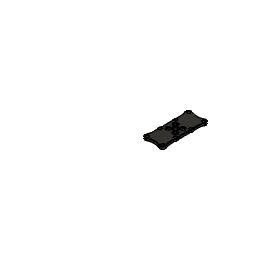
Long BattPad (Autodesk Fusion 360 design; units mm, degrees)
Autodesk Fusion 360 part; units mm, degrees
sketch "Sketch1" plane through (0, 0, 11) normal (0, 0, 1) x (-1, 0, 0)
  circle A0 centre (-10, -10) radius 1.6
  line L0 (-1.822921, 0.176777) -> (-0.176777, 1.822921)
  arc A1 (0.176777, 1.822921) -> (-0.176777, 1.822921) centre (0, 1.646145) ccw
  line L1 (0.176777, 1.822921) -> (1.822921, 0.176777)
  arc A2 (1.822921, -0.176777) -> (1.822921, 0.176777) centre (1.646145, 0) ccw
  line L2 (1.822921, -0.176777) -> (0.176777, -1.822921)
  arc A3 (-0.176777, -1.822921) -> (0.176777, -1.822921) centre (0, -1.646145) ccw
  line L3 (-0.176777, -1.822921) -> (-1.822921, -0.176777)
  arc A4 (-1.822921, 0.176777) -> (-1.822921, -0.176777) centre (-1.646145, 0) ccw
  circle A5 centre (10, 10) radius 1.6
  circle A6 centre (10, -27) radius 1.6
  line L4 (-5.126603, 7.5) -> (-3.5, 7.5)
  arc A7 (-2.5, 6.5) -> (-3.5, 7.5) centre (-3.5, 6.5) ccw
  line L5 (-2.5, 6.5) -> (-2.5, 3.5)
  arc A8 (-3.5, 2.5) -> (-2.5, 3.5) centre (-3.5, 3.5) ccw
  line L6 (-3.5, 2.5) -> (-6.5, 2.5)
  arc A9 (-7.5, 3.5) -> (-6.5, 2.5) centre (-6.5, 3.5) ccw
  line L7 (-7.5, 3.5) -> (-7.5, 5.126603)
  arc A10 (-7.083333, 5.938836) -> (-7.5, 5.126603) centre (-6.5, 5.126603) ccw
  arc A11 (-7.083333, 5.938836) -> (-5.938836, 7.083333) centre (-10, 10) ccw
  arc A12 (-5.126603, 7.5) -> (-5.938836, 7.083333) centre (-5.126603, 6.5) ccw
  circle A13 centre (10, -10) radius 1.6
  circle A14 centre (-10, 10) radius 1.6
  circle A15 centre (-10, -27) radius 1.6
  line L8 (-7.5, -5.126603) -> (-7.5, -3.5)
  arc A16 (-6.5, -2.5) -> (-7.5, -3.5) centre (-6.5, -3.5) ccw
  line L9 (-6.5, -2.5) -> (-3.5, -2.5)
  arc A17 (-2.5, -3.5) -> (-3.5, -2.5) centre (-3.5, -3.5) ccw
  line L10 (-2.5, -3.5) -> (-2.5, -6.5)
  arc A18 (-3.5, -7.5) -> (-2.5, -6.5) centre (-3.5, -6.5) ccw
  line L11 (-3.5, -7.5) -> (-5.126603, -7.5)
  arc A19 (-5.938836, -7.083333) -> (-5.126603, -7.5) centre (-5.126603, -6.5) ccw
  arc A20 (-5.938836, -7.083333) -> (-7.083333, -5.938836) centre (-10, -10) ccw
  arc A21 (-7.5, -5.126603) -> (-7.083333, -5.938836) centre (-6.5, -5.126603) ccw
  circle A22 centre (-10, 27) radius 1.6
  line L12 (5.126603, -7.5) -> (3.5, -7.5)
  arc A23 (2.5, -6.5) -> (3.5, -7.5) centre (3.5, -6.5) ccw
  line L13 (2.5, -6.5) -> (2.5, -3.5)
  arc A24 (3.5, -2.5) -> (2.5, -3.5) centre (3.5, -3.5) ccw
  line L14 (3.5, -2.5) -> (6.5, -2.5)
  arc A25 (7.5, -3.5) -> (6.5, -2.5) centre (6.5, -3.5) ccw
  line L15 (7.5, -3.5) -> (7.5, -5.126603)
  arc A26 (7.083333, -5.938836) -> (7.5, -5.126603) centre (6.5, -5.126603) ccw
  arc A27 (7.083333, -5.938836) -> (5.938836, -7.083333) centre (10, -10) ccw
  arc A28 (5.126603, -7.5) -> (5.938836, -7.083333) centre (5.126603, -6.5) ccw
  line L16 (7.5, 5.126603) -> (7.5, 3.5)
  arc A29 (6.5, 2.5) -> (7.5, 3.5) centre (6.5, 3.5) ccw
  line L17 (6.5, 2.5) -> (3.5, 2.5)
  arc A30 (2.5, 3.5) -> (3.5, 2.5) centre (3.5, 3.5) ccw
  line L18 (2.5, 3.5) -> (2.5, 6.5)
  arc A31 (3.5, 7.5) -> (2.5, 6.5) centre (3.5, 6.5) ccw
  line L19 (3.5, 7.5) -> (5.126603, 7.5)
  arc A32 (5.938836, 7.083333) -> (5.126603, 7.5) centre (5.126603, 6.5) ccw
  arc A33 (5.938836, 7.083333) -> (7.083333, 5.938836) centre (10, 10) ccw
  arc A34 (7.5, 5.126603) -> (7.083333, 5.938836) centre (6.5, 5.126603) ccw
  circle A35 centre (10, 27) radius 1.6
  line L20 (-11.749994, -13.807897) -> (-11.749994, -17.591692)
  arc A36 (-13.425731, -25.474592) -> (-11.749994, -17.591692) centre (-31.128994, -17.591692) ccw
  arc A37 (-13.425731, -25.474592) -> (-8.378659, -30.381383) centre (-10, -27) ccw
  arc A38 (8.378659, -30.381383) -> (-8.378659, -30.381383) centre (0, -47.85547) ccw
  arc A39 (8.378659, -30.381383) -> (13.425731, -25.474592) centre (10, -27) ccw
  arc A40 (11.749994, -17.591692) -> (13.425731, -25.474592) centre (31.128994, -17.591692) ccw
  line L21 (11.749994, -17.591692) -> (11.749994, -13.807897)
  arc A41 (12.395159, -11.351189) -> (11.749994, -13.807897) centre (16.749994, -13.807897) ccw
  arc A42 (12.395159, -11.351189) -> (12.395159, -8.648811) centre (10, -10) ccw
  arc A43 (11.749994, -6.192103) -> (12.395159, -8.648811) centre (16.749994, -6.192103) ccw
  line L22 (11.749994, -6.192103) -> (11.749994, 6.192103)
  arc A44 (12.395159, 8.648811) -> (11.749994, 6.192103) centre (16.749994, 6.192103) ccw
  arc A45 (12.395159, 8.648811) -> (12.395159, 11.351189) centre (10, 10) ccw
  arc A46 (11.749994, 13.807897) -> (12.395159, 11.351189) centre (16.749994, 13.807897) ccw
  line L23 (11.749994, 13.807897) -> (11.749994, 17.591692)
  arc A47 (13.425731, 25.474592) -> (11.749994, 17.591692) centre (31.128994, 17.591692) ccw
  arc A48 (13.425731, 25.474592) -> (8.378659, 30.381383) centre (10, 27) ccw
  arc A49 (-8.378659, 30.381383) -> (8.378659, 30.381383) centre (0, 47.85547) ccw
  arc A50 (-8.378659, 30.381383) -> (-13.425731, 25.474592) centre (-10, 27) ccw
  arc A51 (-11.749994, 17.591692) -> (-13.425731, 25.474592) centre (-31.128994, 17.591692) ccw
  line L24 (-11.749994, 17.591692) -> (-11.749994, 13.807897)
  arc A52 (-12.395159, 11.351189) -> (-11.749994, 13.807897) centre (-16.749994, 13.807897) ccw
  arc A53 (-12.395159, 11.351189) -> (-12.395159, 8.648811) centre (-10, 10) ccw
  arc A54 (-11.749994, 6.192103) -> (-12.395159, 8.648811) centre (-16.749994, 6.192103) ccw
  line L25 (-11.749994, 6.192103) -> (-11.749994, -6.192103)
  arc A55 (-12.395159, -8.648811) -> (-11.749994, -6.192103) centre (-16.749994, -6.192103) ccw
  arc A56 (-12.395159, -8.648811) -> (-12.395159, -11.351189) centre (-10, -10) ccw
  arc A57 (-11.749994, -13.807897) -> (-12.395159, -11.351189) centre (-16.749994, -13.807897) ccw
  arc A58 (-13.06032, -25.637302) -> (-8.551602, -30.020702) centre (-10, -27) ccw
  arc A59 (8.551602, -30.020702) -> (-8.551602, -30.020702) centre (0, -47.85547) ccw
  arc A60 (8.551602, -30.020702) -> (13.06032, -25.637302) centre (10, -27) ccw
  arc A61 (11.349994, -17.591692) -> (13.06032, -25.637302) centre (31.128994, -17.591692) ccw
  line L26 (11.349994, -17.591692) -> (11.349994, -13.807897)
  arc A62 (12.046772, -11.154653) -> (11.349994, -13.807897) centre (16.749994, -13.807897) ccw
  arc A63 (12.046772, -11.154653) -> (12.046772, -8.845347) centre (10, -10) ccw
  arc A64 (11.349994, -6.192103) -> (12.046772, -8.845347) centre (16.749994, -6.192103) ccw
  line L27 (11.349994, -6.192103) -> (11.349994, 6.192103)
  arc A65 (12.046772, 8.845347) -> (11.349994, 6.192103) centre (16.749994, 6.192103) ccw
  arc A66 (12.046772, 8.845347) -> (12.046772, 11.154653) centre (10, 10) ccw
  arc A67 (11.349994, 13.807897) -> (12.046772, 11.154653) centre (16.749994, 13.807897) ccw
  line L28 (11.349994, 13.807897) -> (11.349994, 17.591692)
  arc A68 (13.06032, 25.637302) -> (11.349994, 17.591692) centre (31.128994, 17.591692) ccw
  arc A69 (13.06032, 25.637302) -> (8.551602, 30.020702) centre (10, 27) ccw
  arc A70 (-8.551602, 30.020702) -> (8.551602, 30.020702) centre (0, 47.85547) ccw
  arc A71 (-8.551602, 30.020702) -> (-13.06032, 25.637302) centre (-10, 27) ccw
  arc A72 (-11.349994, 17.591692) -> (-13.06032, 25.637302) centre (-31.128994, 17.591692) ccw
  line L29 (-11.349994, 17.591692) -> (-11.349994, 13.807897)
  arc A73 (-12.046772, 11.154653) -> (-11.349994, 13.807897) centre (-16.749994, 13.807897) ccw
  arc A74 (-12.046772, 11.154653) -> (-12.046772, 8.845347) centre (-10, 10) ccw
  arc A75 (-11.349994, 6.192103) -> (-12.046772, 8.845347) centre (-16.749994, 6.192103) ccw
  line L30 (-11.349994, 6.192103) -> (-11.349994, -6.192103)
  arc A76 (-12.046772, -8.845347) -> (-11.349994, -6.192103) centre (-16.749994, -6.192103) ccw
  arc A77 (-12.046772, -8.845347) -> (-12.046772, -11.154653) centre (-10, -10) ccw
  arc A78 (-11.349994, -13.807897) -> (-12.046772, -11.154653) centre (-16.749994, -13.807897) ccw
  line L31 (-11.349994, -13.807897) -> (-11.349994, -17.591692)
  arc A79 (-13.06032, -25.637302) -> (-11.349994, -17.591692) centre (-31.128994, -17.591692) ccw
  circle A80 centre (-10, 10) radius 1.8
  circle A81 centre (10, 10) radius 1.8
  circle A82 centre (10, -10) radius 1.8
  circle A83 centre (10, -27) radius 1.8
  circle A84 centre (-10, -27) radius 1.8
  circle A85 centre (-10, 27) radius 1.8
  circle A86 centre (10, 27) radius 1.8
  dimension "d510" = 0.4
  dimension "d511" = 0.2
  dimension "d512" = 0.2
  dimension "d513" = 0.2
  dimension "d514" = 0.2
  dimension "d515" = 0.2
  dimension "d516" = 0.2
  dimension "d517" = 0.2
extrude "Extrude1" add sketch "Sketch1" along normal blind 3 contours A58 A59 A60 A61 L26 A62 A63 A64 L27 A65 A66 A67 L28 A68 A69 A70 A71 A72 L29 A73 A74 A75 L30 A76 A77 A78 L31 A79 picked at (0, 14.331819)
fillet "Fillet1" radius 0.336 28 edges at (11.7823, -21.704388, 14) (11.349994, -15.699795, 14) (11.527093, -12.436292, 14) (12.35, -10, 14) (11.527093, -7.563708, 14) (11.349994, 0, 14) (11.527093, 7.563708, 14) (12.35, 10, 14) (11.527093, 12.436292, 14) (11.349994, 15.699795, 14) (11.7823, 21.704388, 14) (12.335192, 29.401953, 14) (0, 28.07647, 14) (-12.335192, 29.401953, 14) (-11.7823, 21.704388, 14) (-11.349994, 15.699795, 14) (-11.527093, 12.436292, 14) (-12.35, 10, 14) (-11.527093, 7.563708, 14) (-11.349994, 0, 14) (-11.527093, -7.563708, 14) (-12.35, -10, 14) (-11.527093, -12.436292, 14) (-11.349994, -15.699795, 14) (-11.7823, -21.704388, 14) (-12.335192, -29.401953, 14) (0, -28.07647, 14) (12.335192, -29.401953, 14)
fillet "Fillet2" radius 0.4 56 edges at (4.313301, 7.5, 14) (5.583038, 7.389757, 14) (6.464466, 6.464466, 14) (7.389757, 5.583038, 14) (7.5, 4.313301, 14) (7.207107, 2.792893, 14) (5, 2.5, 14) (2.792893, 2.792893, 14) (2.5, 5, 14) (2.792893, 7.207107, 14) (7.5, -4.313301, 14) (7.389757, -5.583038, 14) (6.464466, -6.464466, 14) (5.583038, -7.389757, 14) (4.313301, -7.5, 14) (2.792893, -7.207107, 14) (2.5, -5, 14) (2.792893, -2.792893, 14) (5, -2.5, 14) (7.207107, -2.792893, 14) (0, -1.896145, 14) (-0.999849, -0.999849, 14) (-1.896145, 0, 14) (-0.999849, 0.999849, 14) (0, 1.896145, 14) (0.999849, 0.999849, 14) (1.896145, 0, 14) (0.999849, -0.999849, 14) (-2.792893, -7.207107, 14) (-4.313301, -7.5, 14) (-5.583038, -7.389757, 14) (-6.464466, -6.464466, 14) (-7.389757, -5.583038, 14) (-7.5, -4.313301, 14) (-7.207107, -2.792893, 14) (-5, -2.5, 14) (-2.792893, -2.792893, 14) (-2.5, -5, 14) (-7.5, 4.313301, 14) (-7.389757, 5.583038, 14) (-6.464466, 6.464466, 14) (-5.583038, 7.389757, 14) (-4.313301, 7.5, 14) (-2.792893, 7.207107, 14) (-2.5, 5, 14) (-2.792893, 2.792893, 14) (-5, 2.5, 14) (-7.207107, 2.792893, 14) (-8.321811, 9.349092, 14) (-8.321811, -10.650908, 14) (11.678189, -10.650908, 14) (11.678189, -27.650908, 14) (-8.321811, -27.650908, 14) (11.678189, 26.349092, 14) (11.491724, 9.421415, 14) (-8.321811, 26.349092, 14)
sketch "Sketch1 (1)" plane through (0, 0, 14) normal (0, 0, 1) x (-1, 0, 0)
  circle A0 centre (-10, -10) radius 2
  circle A1 centre (10, 27) radius 2.2
  arc A2 (-11.424764, 8.323681) -> (-11.424764, 11.676319) centre (-10, 10) ccw
  arc A3 (-11.013994, 6.192103) -> (-11.424764, 8.323681) centre (-16.749994, 6.192103) ccw
  line L0 (-11.013994, 6.192103) -> (-11.013994, -6.192103)
  arc A4 (-11.754127, -9.010438) -> (-11.013994, -6.192103) centre (-16.749994, -6.192103) ccw
  arc A5 (-11.754127, -9.010438) -> (-11.754127, -10.989562) centre (-10, -10) ccw
  arc A6 (-11.013994, -13.807897) -> (-11.754127, -10.989562) centre (-16.749994, -13.807897) ccw
  line L1 (-11.013994, -13.807897) -> (-11.013994, -17.591692)
  arc A7 (-12.753374, -25.773979) -> (-11.013994, -17.591692) centre (-31.128994, -17.591692) ccw
  arc A8 (-12.753374, -25.773979) -> (-8.696874, -29.71773) centre (-10, -27) ccw
  arc A9 (8.696874, -29.71773) -> (-8.696874, -29.71773) centre (0, -47.85547) ccw
  arc A10 (8.696874, -29.71773) -> (12.753374, -25.773979) centre (10, -27) ccw
  arc A11 (11.013994, -17.591692) -> (12.753374, -25.773979) centre (31.128994, -17.591692) ccw
  line L2 (11.013994, -17.591692) -> (11.013994, -13.807897)
  arc A12 (11.424764, -11.676319) -> (11.013994, -13.807897) centre (16.749994, -13.807897) ccw
  arc A13 (11.424764, -8.323681) -> (11.424764, -11.676319) centre (10, -10) ccw
  arc A14 (11.013994, -6.192103) -> (11.424764, -8.323681) centre (16.749994, -6.192103) ccw
  line L3 (11.013994, -6.192103) -> (11.013994, 6.192103)
  arc A15 (11.424764, 8.323681) -> (11.013994, 6.192103) centre (16.749994, 6.192103) ccw
  arc A16 (11.424764, 11.676319) -> (11.424764, 8.323681) centre (10, 10) ccw
  arc A17 (11.013994, 13.807897) -> (11.424764, 11.676319) centre (16.749994, 13.807897) ccw
  line L4 (11.013994, 13.807897) -> (11.013994, 17.591692)
  arc A18 (12.753374, 25.773979) -> (11.013994, 17.591692) centre (31.128994, 17.591692) ccw
  arc A19 (12.753374, 25.773979) -> (8.696874, 29.71773) centre (10, 27) ccw
  arc A20 (-8.696874, 29.71773) -> (8.696874, 29.71773) centre (0, 47.85547) ccw
  arc A21 (-8.696874, 29.71773) -> (-12.753374, 25.773979) centre (-10, 27) ccw
  arc A22 (-11.013994, 17.591692) -> (-12.753374, 25.773979) centre (-31.128994, 17.591692) ccw
  line L5 (-11.013994, 17.591692) -> (-11.013994, 13.807897)
  arc A23 (-11.424764, 11.676319) -> (-11.013994, 13.807897) centre (-16.749994, 13.807897) ccw
  arc A24 (3.5, 7.9) -> (2.1, 6.5) centre (3.5, 6.5) ccw
  line L6 (3.5, 7.9) -> (5.126603, 7.9)
  arc A25 (6.263729, 7.316667) -> (5.126603, 7.9) centre (5.126603, 6.5) ccw
  arc A26 (6.263729, 7.316667) -> (7.316667, 6.263729) centre (10, 10) ccw
  arc A27 (7.9, 5.126603) -> (7.316667, 6.263729) centre (6.5, 5.126603) ccw
  line L7 (7.9, 5.126603) -> (7.9, 3.5)
  arc A28 (6.5, 2.1) -> (7.9, 3.5) centre (6.5, 3.5) ccw
  line L8 (6.5, 2.1) -> (3.5, 2.1)
  arc A29 (2.1, 3.5) -> (3.5, 2.1) centre (3.5, 3.5) ccw
  line L9 (2.1, 3.5) -> (2.1, 6.5)
  line L10 (-7.9, 3.5) -> (-7.9, 5.126603)
  arc A30 (-7.316667, 6.263729) -> (-7.9, 5.126603) centre (-6.5, 5.126603) ccw
  arc A31 (-7.316667, 6.263729) -> (-6.263729, 7.316667) centre (-10, 10) ccw
  arc A32 (-5.126603, 7.9) -> (-6.263729, 7.316667) centre (-5.126603, 6.5) ccw
  line L11 (-5.126603, 7.9) -> (-3.5, 7.9)
  arc A33 (-2.1, 6.5) -> (-3.5, 7.9) centre (-3.5, 6.5) ccw
  line L12 (-2.1, 6.5) -> (-2.1, 3.5)
  arc A34 (-3.5, 2.1) -> (-2.1, 3.5) centre (-3.5, 3.5) ccw
  line L13 (-3.5, 2.1) -> (-6.5, 2.1)
  arc A35 (-7.9, 3.5) -> (-6.5, 2.1) centre (-6.5, 3.5) ccw
  line L14 (-3.5, -7.9) -> (-5.126603, -7.9)
  arc A36 (-6.263729, -7.316667) -> (-5.126603, -7.9) centre (-5.126603, -6.5) ccw
  arc A37 (-6.263729, -7.316667) -> (-7.316667, -6.263729) centre (-10, -10) ccw
  arc A38 (-7.9, -5.126603) -> (-7.316667, -6.263729) centre (-6.5, -5.126603) ccw
  line L15 (-7.9, -5.126603) -> (-7.9, -3.5)
  arc A39 (-6.5, -2.1) -> (-7.9, -3.5) centre (-6.5, -3.5) ccw
  line L16 (-6.5, -2.1) -> (-3.5, -2.1)
  arc A40 (-2.1, -3.5) -> (-3.5, -2.1) centre (-3.5, -3.5) ccw
  line L17 (-2.1, -3.5) -> (-2.1, -6.5)
  arc A41 (-3.5, -7.9) -> (-2.1, -6.5) centre (-3.5, -6.5) ccw
  arc A42 (0.459619, 2.105764) -> (-0.459619, 2.105764) centre (0, 1.646145) ccw
  line L18 (0.459619, 2.105764) -> (2.105764, 0.459619)
  arc A43 (2.105764, -0.459619) -> (2.105764, 0.459619) centre (1.646145, 0) ccw
  line L19 (2.105764, -0.459619) -> (0.459619, -2.105764)
  arc A44 (-0.459619, -2.105764) -> (0.459619, -2.105764) centre (0, -1.646145) ccw
  line L20 (-0.459619, -2.105764) -> (-2.105764, -0.459619)
  arc A45 (-2.105764, 0.459619) -> (-2.105764, -0.459619) centre (-1.646145, 0) ccw
  line L21 (-2.105764, 0.459619) -> (-0.459619, 2.105764)
  line L22 (7.9, -3.5) -> (7.9, -5.126603)
  arc A46 (7.316667, -6.263729) -> (7.9, -5.126603) centre (6.5, -5.126603) ccw
  arc A47 (7.316667, -6.263729) -> (6.263729, -7.316667) centre (10, -10) ccw
  arc A48 (5.126603, -7.9) -> (6.263729, -7.316667) centre (5.126603, -6.5) ccw
  line L23 (5.126603, -7.9) -> (3.5, -7.9)
  arc A49 (2.1, -6.5) -> (3.5, -7.9) centre (3.5, -6.5) ccw
  line L24 (2.1, -6.5) -> (2.1, -3.5)
  arc A50 (3.5, -2.1) -> (2.1, -3.5) centre (3.5, -3.5) ccw
  line L25 (3.5, -2.1) -> (6.5, -2.1)
  arc A51 (7.9, -3.5) -> (6.5, -2.1) centre (6.5, -3.5) ccw
  circle A52 centre (-10, 27) radius 2.2
  circle A53 centre (-10, -27) radius 2.2
  circle A54 centre (10, -27) radius 2.2
  arc A55 (0.792893, -3.262742) -> (1.146447, -3.116295) centre (0.792893, -2.762742) ccw
  line L26 (1.146447, -3.116295) -> (3.116295, -1.146447)
  arc A56 (3.116295, -1.146447) -> (3.262742, -0.792893) centre (2.762742, -0.792893) ccw
  line L27 (3.262742, -0.792893) -> (3.262742, 0.792893)
  arc A57 (3.262742, 0.792893) -> (3.116295, 1.146447) centre (2.762742, 0.792893) ccw
  line L28 (3.116295, 1.146447) -> (1.146447, 3.116295)
  arc A58 (1.146447, 3.116295) -> (0.792893, 3.262742) centre (0.792893, 2.762742) ccw
  line L29 (0.792893, 3.262742) -> (-0.792893, 3.262742)
  arc A59 (-0.792893, 3.262742) -> (-1.146447, 3.116295) centre (-0.792893, 2.762742) ccw
  line L30 (-1.146447, 3.116295) -> (-3.116295, 1.146447)
  arc A60 (-3.116295, 1.146447) -> (-3.262742, 0.792893) centre (-2.762742, 0.792893) ccw
  line L31 (-3.262742, 0.792893) -> (-3.262742, -0.792893)
  arc A61 (-3.262742, -0.792893) -> (-3.116295, -1.146447) centre (-2.762742, -0.792893) ccw
  line L32 (-3.116295, -1.146447) -> (-1.146447, -3.116295)
  arc A62 (-1.146447, -3.116295) -> (-0.792893, -3.262742) centre (-0.792893, -2.762742) ccw
  line L33 (-0.792893, -3.262742) -> (0.792893, -3.262742)
  line L34 (3.292742, -0.792893) -> (3.292742, 0.792893)
  arc A63 (3.292742, 0.792893) -> (3.137508, 1.16766) centre (2.762742, 0.792893) ccw
  line L35 (3.137508, 1.16766) -> (1.16766, 3.137508)
  arc A64 (1.16766, 3.137508) -> (0.792893, 3.292742) centre (0.792893, 2.762742) ccw
  line L36 (0.792893, 3.292742) -> (-0.792893, 3.292742)
  arc A65 (-0.792893, 3.292742) -> (-1.16766, 3.137508) centre (-0.792893, 2.762742) ccw
  line L37 (-1.16766, 3.137508) -> (-3.137508, 1.16766)
  arc A66 (-3.137508, 1.16766) -> (-3.292742, 0.792893) centre (-2.762742, 0.792893) ccw
  line L38 (-3.292742, 0.792893) -> (-3.292742, -0.792893)
  arc A67 (-3.292742, -0.792893) -> (-3.137508, -1.16766) centre (-2.762742, -0.792893) ccw
  line L39 (-3.137508, -1.16766) -> (-1.16766, -3.137508)
  arc A68 (-1.16766, -3.137508) -> (-0.792893, -3.292742) centre (-0.792893, -2.762742) ccw
  line L40 (-0.792893, -3.292742) -> (0.792893, -3.292742)
  arc A69 (0.792893, -3.292742) -> (1.16766, -3.137508) centre (0.792893, -2.762742) ccw
  line L41 (1.16766, -3.137508) -> (3.137508, -1.16766)
  arc A70 (3.137508, -1.16766) -> (3.292742, -0.792893) centre (2.762742, -0.792893) ccw
  dimension "d584" = 0.03
extrude "Extrude2" cut sketch "Sketch1 (1)" against normal up to surface (11.5 mm away) contours A42 L18 A43 L19 A44 L20 A45 L21 | A55 L26 A56 L27 A57 L28 A58 L29 A59 L30 A60 L31 A61 L32 A62 L33 picked at (-0.701921, 0.153206) picked at (1.57412, 2.122835)
fillet "Fillet3" radius 0.4 16 edges at (-3.262742, 0, 14) (-3.224681, 0.984235, 14) (-2.131371, 2.131371, 14) (-0.984235, 3.224681, 14) (0, 3.262742, 14) (0.984235, 3.224681, 14) (2.131371, 2.131371, 14) (3.224681, 0.984235, 14) (3.262742, 0, 14) (3.224681, -0.984235, 14) (2.131371, -2.131371, 14) (0.984235, -3.224681, 14) (0, -3.262742, 14) (-0.984235, -3.224681, 14) (-2.131371, -2.131371, 14) (-3.224681, -0.984235, 14)
